dog lid (Autodesk Fusion 360 design; units mm, degrees)
Autodesk Fusion 360 part; units mm, degrees
sketch "Sketch1" plane through (0, 0, 0) normal (0, 0, 1) x (1, 0, 0)
  circle A0 centre (0, 0) radius 51
  circle A1 centre (0, 0) radius 48.75
  circle A2 centre (0, 0) radius 52
  circle A3 centre (0, 0) radius 46.75
  circle A4 centre (0, 0) radius 50.5
  dimension "d1" = 102
  dimension "d2" = 97.5
  dimension "d3" = 104
  dimension "d6" = 93.5
  dimension "d11" = 101
  constraint coincident A0.centre A1.centre
  constraint concentric A0 A1
  constraint concentric A0 A2
  constraint concentric A0 A3
  measures "d1" diameter of A0
  measures "d2" diameter of A1
  measures "d3" diameter of A2
  measures "d6" diameter of A3
  measures "d11" diameter of A4
extrude "Extrude1" add sketch "Sketch1" along normal blind 0.6 contours A0 | A1 | A2 | A3 | A4
extrude "Extrude3" add sketch "Sketch1" along normal blind 4.26 contours A2
extrude "Extrude4" add sketch "Sketch1" along normal blind 1 from surface at 3.26 contours A0
fillet "Fillet1" radius 0.75 1 edges at (-47.5487, -18.4424, 3.26)
equation "d1 = size"
equation "d2 = size - 4.5 mm"
equation "d3 = size + 2 mm"
equation "d4 = thickness"
equation "d6 = size - 8.5 mm"
equation "d9 = thickness + overhang + chamber"
equation "d11 = size - 1 mm"
equation "d12 = thickness + chamber"
equation "d13 = overhang"
equation "size = 102 mm"
equation "thickness = 0.6 mm"
equation "overhang = 1 mm"
equation "chamber = 2.66 mm"
